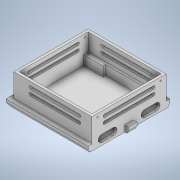
# Autodesk Inventor part: GameFrameRaspiBox1
Saved by Autodesk Inventor 2022 (Build 260153000, 153)
## iProperties
Created: 2022-03-27
Part Number: GameFrameRaspiBox1
Material: Generisch
Document SubType Name: Modeling
Designer: Max
Density: 1 g/cm^3
Appearance: Vorgabe
Author: Max
Autodesk Inventor part; units mm, degrees
ref_plane "YZ Plane" through (0, 0, 0) normal (1, 0, 0) x (0, 1, 0)
ref_plane "XZ Plane" through (0, 0, 0) normal (0, 1, 0) x (-1, 0, 0)
ref_plane "XY Plane" through (0, 0, 0) normal (0, 0, 1) x (1, 0, 0)
sketch "Skizze1" plane through (0, 0, 0) normal (0, 1, 0) x (-1, 0, 0)
  line L0 (16.4314, 33.2132) -> (-63.5686, 33.2132)
  line L1 (-63.5686, 33.2132) -> (-63.5686, -42.7868)
  line L2 (-63.5686, -42.7868) -> (16.4314, -42.7868)
  line L3 (16.4314, -42.7868) -> (16.4314, 33.2132)
  point P0 (0, 0)
  dimension "d0" = 76
  dimension "d1" = 80
  constraints: 8 end point, 2 parallel, 1 horizontal, 1 perpendicular
  measures "d0" distance of L2.end L0.start
  measures "d1" distance of L0.start L0.end
extrude "Extrusion1" add sketch "Skizze1" along normal blind 30.5
shell "Wandung1" thickness 2.5 removed faces 1 at (36.9019, 30.5, 7.8799)
sketch "Skizze2" plane through (-13.9314, 2.5, -40.2868) normal (0, 1, 0) x (1, 0, 0)
  line L0 (0, -71) -> (0, 0) projected
  line L1 (75, 0) -> (75, -71) projected
  line L2 (75, -71) -> (75, 0) projected
  line L3 (0, 0) -> (0, -71) projected
  line L4 (0, -71) -> (0, -66.5)
  line L5 (0, -66.5) -> (20, -66.5)
  line L6 (20, -66.5) -> (20, -69)
  line L7 (20, -69) -> (75, -69)
  line L8 (75, -69) -> (75, -71)
  line L9 (0, -71) -> (75, -71) projected
  line L10 (0, -35.5) -> (75, -35.5)
  line L11 (0, 0) -> (0, -4.5)
  line L12 (0, -4.5) -> (20, -4.5)
  line L13 (20, -4.5) -> (20, -2)
  line L14 (20, -2) -> (75, -2)
  line L15 (75, -2) -> (75, 0)
  line L16 (0, 0) -> (75, 0)
  point P0 (75, 0)
  point P1 (75, -2)
  point P2 (0, -4.5)
  point P3 (0, -66.5)
  dimension "d35" = 4.5
  dimension "d36" = 2
  dimension "d37" = 20
  constraints: 24 end point, 7 symmetric about line, 4 point on line, 3 perpendicular, 2 midpoint, 1 horizontal
  measures "d35" distance between parallel lines of L9 L5
  measures "d36" distance of L7.end L8.end
  measures "d37" distance between parallel lines of L6 L0
extrude "Extrusion2" add sketch "Skizze2" along normal blind 10 contours L0 L5 L6 L7 L1 L9 | L0 L16 L1 L14 L13 L12
sketch "Skizze3" plane through (-13.9314, 12.5, -40.2868) normal (0, 1, 0) x (1, 0, 0)
  circle A0 centre (2.25, -68.75) radius 0.75
  line L0 (2.25, -68.75) -> (2.25, -66.5) construction
  line L1 (2.25, -68.75) -> (0, -68.75) construction
  line L2 (0, -71) -> (0, 0) construction
  line L3 (75, 0) -> (75, -71) construction
  line L4 (75, -71) -> (0, -71) construction
  circle A1 centre (2.25, -2.25) radius 0.75
  line L5 (0, 0) -> (75, 0) projected
  point P0 (13.9314, -40.2868)
  dimension "d8" = 1.5
  dimension "d14" = 2.25
  dimension "d38" = 2.25
  dimension "d39" = 2.25
  dimension "d40" = 2.25
  constraints: 4 end point, 2 centre point, 1 equal radius, 1 perpendicular, 1 point on line, 1 vertical
  measures "d8" diameter of A0
  measures "d14" distance of L0.start L1.end
  measures "d38" distance from line of L4 L0.start
  measures "d39" distance from line of L2 A1.centre
  measures "d40" distance from line of L5 A1.centre
extrude "Extrusion3" cut sketch "Skizze3" against normal blind 8
sketch "Skizze6" plane through (63.5686, 0, 33.2132) normal (1, 0, 0) x (0, 0, -1)
  line L0 (69.5, 10) -> (69.5, 2.75)
  line L1 (0, 0) -> (76, 0) projected
  line L2 (76, 0) -> (76, 30.5) projected
  line L3 (0, 0) -> (0, 30.5) projected
  line L4 (10, 6.375) -> (22, 6.375) construction
  line L5 (10, 2.75) -> (22, 2.75)
  line L6 (22, 10) -> (10, 10)
  arc A0 (10, 10) -> (10, 2.75) centre (10, 6.375) ccw
  arc A1 (22, 2.75) -> (22, 10) centre (22, 6.375) ccw
  line L7 (54, 6.375) -> (66, 6.375) construction
  line L8 (54, 2.75) -> (66, 2.75)
  line L9 (66, 10) -> (54, 10)
  arc A2 (54, 10) -> (54, 2.75) centre (54, 6.375) ccw
  arc A3 (66, 2.75) -> (66, 10) centre (66, 6.375) ccw
  point P0 (33.2132, 0)
  point P1 (16, 6.375)
  point P2 (60, 6.375)
  point P3 (69.5, 5.4313)
  point P4 (69.5, 7.3187)
  dimension "d31" = 6.5
  dimension "d59" = 7.25
  dimension "d60" = 2.75
  dimension "d61" = 10
  dimension "d62" = 12
  dimension "d63" = 7.25
  dimension "d64" = 12
  dimension "d65" = 2.75
  dimension "d66" = 10
  constraints: 18 end point, 8 point on circle, 8 tangent, 4 centre point, 2 horizontal, 2 midpoint, 2 parallel
  measures "d31" distance between parallel lines of L2 L0
  measures "d59" distance between parallel lines of L5 L6
  measures "d60" distance between parallel lines of L1 L5
  measures "d61" distance from line of L3 L4.start
  measures "d62" distance of L6.start L6.end
  measures "d63" distance between parallel lines of L8 L9
  measures "d64" distance of L9.start L9.end
  measures "d65" distance between parallel lines of L1 L8
  measures "d66" distance from line of L2 L7.end
extrude "Extrusion6" cut sketch "Skizze6" against normal blind 10 contours L0 A3 L8 A2 L9 | A0 L6 A1 L5
sketch "Skizze8" plane through (-13.9314, 30.5, 30.7132) normal (1, 0, 0) x (0, 0, -1)
  circle A0 centre (3.2, -3.25) radius 0.75
  circle A1 centre (67.8, -3.25) radius 0.75
  line L0 (0, -18) -> (0, 0) projected
  line L1 (0, 0) -> (71, 0) projected
  line L2 (71, -18) -> (71, 0) projected
  line L3 (10.5, -5.5) -> (60.5, -5.5) construction
  line L4 (10.5, -4) -> (60.5, -4)
  line L5 (60.5, -7) -> (10.5, -7)
  arc A2 (10.5, -4) -> (10.5, -7) centre (10.5, -5.5) ccw
  arc A3 (60.5, -7) -> (60.5, -4) centre (60.5, -5.5) ccw
  line L6 (10.5, -11.5) -> (60.5, -11.5) construction
  line L7 (10.5, -10) -> (60.5, -10)
  line L8 (60.5, -13) -> (10.5, -13)
  arc A4 (10.5, -10) -> (10.5, -13) centre (10.5, -11.5) ccw
  arc A5 (60.5, -13) -> (60.5, -10) centre (60.5, -11.5) ccw
  point P0 (30.7132, -30.5)
  point P1 (35.5, -5.5)
  point P2 (35.5, -11.5)
  dimension "d43" = 1.5
  dimension "d44" = 3.2
  dimension "d45" = 3.25
  dimension "d46" = 3.2
  dimension "d47" = 3.25
  dimension "d50" = 3
  dimension "d51" = 4
  dimension "d53" = 50
  dimension "d54" = 3
  dimension "d55" = 50
  dimension "d56" = 35.5
  dimension "d57" = 3
  dimension "d58" = 35.5
  constraints: 16 end point, 8 point on circle, 8 tangent, 6 centre point, 3 parallel, 2 midpoint, 1 equal radius
  measures "d43" diameter of A0
  measures "d44" distance from line of L0 A0.centre
  measures "d45" distance from line of L1 A0.centre
  measures "d46" distance from line of L2 A1.centre
  measures "d47" distance from line of L1 A1.centre
  measures "d50" distance between parallel lines of L5 L4
  measures "d51" distance between parallel lines of L1 L4
  measures "d53" distance of L4.start L4.end
  measures "d54" distance between parallel lines of L8 L7
  measures "d55" distance of L7.start L7.end
  measures "d56" distance from line of L0 point (35.5, -5.5)
  measures "d57" distance between parallel lines of L5 L7
  measures "d58" distance from line of L0 point (35.5, -11.5)
extrude "Extrusion7" cut sketch "Skizze8" along normal through all both and the other way through all
sketch "Skizze9" plane through (61.0686, 30.5, 30.7132) normal (0, 0, -1) x (-1, 0, 0)
  line L0 (10.5, -5.5) -> (60.5, -5.5) construction
  line L1 (77.5, 0) -> (-2.5, 0) projected
  line L2 (10.5, -4) -> (60.5, -4)
  line L3 (60.5, -7) -> (10.5, -7)
  arc A0 (10.5, -4) -> (10.5, -7) centre (10.5, -5.5) ccw
  arc A1 (60.5, -7) -> (60.5, -4) centre (60.5, -5.5) ccw
  line L4 (0, -18) -> (0, 0) projected
  line L5 (10.5, -11.5) -> (60.5, -11.5) construction
  line L6 (10.5, -10) -> (60.5, -10)
  line L7 (60.5, -13) -> (10.5, -13)
  arc A2 (10.5, -10) -> (10.5, -13) centre (10.5, -11.5) ccw
  arc A3 (60.5, -13) -> (60.5, -10) centre (60.5, -11.5) ccw
  point P0 (61.0686, -30.5)
  point P1 (35.5, -5.5)
  point P2 (35.5, -11.5)
  dimension "d67" = 50
  dimension "d68" = 35.5
  dimension "d69" = 3
  dimension "d70" = 4
  dimension "d71" = 50
  dimension "d72" = 3
  dimension "d73" = 35.5
  dimension "d74" = 3
  constraints: 16 end point, 8 point on circle, 8 tangent, 4 centre point, 3 parallel, 2 midpoint
  measures "d67" distance of L2.start L2.end
  measures "d68" distance from line of L4 point (35.5, -5.5)
  measures "d69" distance between parallel lines of L3 L2
  measures "d70" distance between parallel lines of L1 L2
  measures "d71" distance of L6.start L6.end
  measures "d72" distance between parallel lines of L7 L6
  measures "d73" distance from line of L4 point (35.5, -11.5)
  measures "d74" distance between parallel lines of L3 L6
extrude "Extrusion8" cut sketch "Skizze9" along normal through all both and the other way through all
sketch "Skizze10" plane through (-16.4314, 0, 33.2132) normal (0, 0, 1) x (1, 0, 0)
  line L0 (0, 0) -> (0, 30.5) projected
  line L1 (80, 0) -> (0, 0)
  line L2 (0, 0) -> (0, 6.5)
  line L3 (0, 6.5) -> (80, 6.5)
  line L4 (80, 6.5) -> (80, 0)
  point P0 (16.4314, 0)
  dimension "d77" = 6.5
  constraints: 8 end point, 2 parallel, 1 horizontal, 1 perpendicular, 1 point on line
  measures "d77" distance between parallel lines of L1 L3
extrude "Extrusion9" add sketch "Skizze10" along normal blind 4
sketch "Skizze11" plane through (63.5686, 0, -42.7868) normal (0, 0, -1) x (-1, 0, 0)
  line L0 (0, 0) -> (0, 30.5) projected
  line L1 (80, 0) -> (80, 30.5) projected
  line L2 (0, 0) -> (80, 0)
  line L3 (80, 0) -> (80, 6.5)
  line L4 (80, 6.5) -> (0, 6.5)
  line L5 (0, 6.5) -> (0, 0)
  point P0 (63.5686, 0)
  point P1 (0, 6.5)
  dimension "d80" = 6.5
  constraints: 8 end point, 2 parallel, 1 horizontal, 1 perpendicular, 1 point on line
  measures "d80" distance between parallel lines of L2 L4
extrude "Extrusion10" add sketch "Skizze11" along normal blind 4
sketch "Skizze12" plane through (-16.4314, 30.5, -42.7868) normal (-1, 0, 0) x (0, 0, 1)
  line L0 (80, -30.5) -> (-4, -30.5) projected
  line L1 (76, -24) -> (80, -24) projected
  line L2 (-4, -30.5) -> (80, -30.5)
  line L3 (80, -30.5) -> (80, -24)
  line L4 (80, -24) -> (-4, -24)
  line L5 (-4, -24) -> (-4, -30.5)
  point P0 (42.7868, -30.5)
  constraints: 8 end point, 2 parallel, 1 horizontal, 1 perpendicular
extrude "Extrusion11" add sketch "Skizze12" along normal blind 4
sketch "Skizze13" plane through (63.5686, 30.5, 33.2132) normal (1, 0, 0) x (0, 0, -1)
  line L0 (33.625, -24) -> (42.375, -24)
  line L1 (42.375, -24) -> (42.375, -30.5)
  line L2 (42.375, -30.5) -> (33.625, -30.5)
  line L3 (33.625, -30.5) -> (33.625, -24)
  line L4 (-4, -30.5) -> (80, -30.5) projected
  arc A0 (22, -27.75) -> (22, -20.5) centre (22, -24.125) ccw projected
  point P0 (33.2132, -30.5)
  dimension "d85" = 6.5
  dimension "d86" = 8.75
  dimension "d87" = 15.25
  constraints: 8 end point, 2 parallel, 1 horizontal, 1 perpendicular, 1 point on line
  measures "d85" distance between parallel lines of L2 L0
  measures "d86" distance of L0.start L0.end
extrude "Extrusion12" add sketch "Skizze13" along normal blind 4
chamfer "Fase1" distance 2 angle 60 4 edges at (21.5686, 0, 37.2132) (-20.4314, 0, -4.7868) (21.5686, 0, -46.7868) (67.5686, 0, -4.7868) measured on face at (7.5686, 0, -3.3285)
